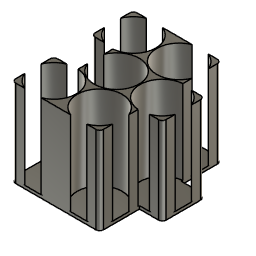
Plate_Holder (Autodesk Fusion 360 design; units mm, degrees)
Autodesk Fusion 360 part; units mm, degrees
note: some values were not read from the file. Set by a fixed rule: which sketch regions a step uses.
sketch "Sketch4" plane through (0, 0, 0) normal (0, 0, 1) x (1, 0, 0)
  circle A0 centre (-30.1021, 33.9333) radius 30
  circle A1 centre (30.8979, 33.9333) radius 30
  circle A2 centre (0.3979, -19.0667) radius 30
  circle A3 centre (-60.6021, -19.0667) radius 30
  line L0 (-84.1021, 5.9333) -> (-84.1021, 6.9333)
  line L1 (27.3979, -43.0667) -> (26.9, -43.0667)
  circle A4 centre (0.3979, 86.9333) radius 30
  circle A5 centre (-60.6021, 86.9333) radius 30
  line L2 (-88.6021, 114.9333) -> (58.8979, 114.9333)
  line L3 (58.8979, 114.9333) -> (58.8979, -47.0667)
  line L4 (58.8979, -47.0667) -> (-88.6021, -47.0667)
  line L5 (-88.6021, -47.0667) -> (-88.6021, 114.9333)
  line L6 (-88.6021, 58.9333) -> (-58.1021, 58.9333)
  line L7 (-58.1021, 58.9333) -> (-58.1021, 8.9333)
  line L8 (-58.1021, 8.9333) -> (-88.6021, 8.9333)
  line L9 (-88.6021, 8.9333) -> (-88.6021, 58.9333)
  line L10 (58.8979, 61.9333) -> (28.3979, 61.9333)
  line L11 (28.3979, 61.9333) -> (28.3979, 114.9333)
  line L12 (28.3979, 114.9333) -> (58.8979, 114.9333)
  line L13 (58.8979, 114.9333) -> (58.8979, 61.9333)
  line L14 (58.8979, 5.9333) -> (28.3979, 5.9333)
  line L15 (28.3979, 5.9333) -> (28.3979, -47.0667)
  line L16 (28.3979, -47.0667) -> (58.8979, -47.0667)
  line L17 (58.8979, -47.0667) -> (58.8979, 5.9333)
  dimension "d15" = 60
  dimension "d16" = 60
  dimension "d17" = 60
  dimension "d18" = 60
  dimension "d19" = 61
  dimension "d23" = 61
  dimension "d24" = 30.5
  dimension "d25" = 53
  dimension "d46" = 60
  dimension "d47" = 60
  dimension "d48" = 61
  dimension "d49" = 53
  dimension "d50" = 30.5
  dimension "d53" = 28
  dimension "d54" = 28
  dimension "d55" = 28
  dimension "d56" = 28
  dimension "d57" = 28
  dimension "d58" = 28
  dimension "d59" = 28
  dimension "d60" = 28
  dimension "d61" = 28
  dimension "d62" = 28
  dimension "d63" = 28
  dimension "d64" = 28
  constraint vertical L0
  constraint horizontal L1
  constraint horizontal L2
  constraint vertical L3
  constraint horizontal L4
  constraint vertical L5
  constraint horizontal L6
  constraint vertical L7
  constraint horizontal L8
  constraint vertical L9
  constraint coincident L5 L6.start
  constraint horizontal L10
  constraint vertical L11
  constraint horizontal L12
  constraint vertical L13
  constraint coincident L2 L11.end
  constraint coincident L3 L10.start
  constraint horizontal L14
  constraint vertical L15
  constraint horizontal L16
  constraint vertical L17
  constraint coincident L4 L15.end
  constraint coincident L3 L14.start
  measures "d15" diameter of A3
  measures "d16" diameter of A2
  measures "d17" diameter of A1
  measures "d18" diameter of A0
  measures "d19" distance of A0.centre A1.centre
  measures "d23" horizontal distance of A2.centre A3.centre
  measures "d24" horizontal distance of A1.centre A2.centre
  measures "d25" vertical distance of A1.centre A2.centre
  measures "d46" diameter of A5
  measures "d47" diameter of A4
  measures "d48" distance of A4.centre A5.centre
  measures "d49" vertical distance of A1.centre A4.centre
  measures "d50" horizontal distance of A1.centre A4.centre
  measures "d53" distance of A2.centre L4
  measures "d54" distance of A4.centre L2
  measures "d55" distance of A5.centre L5
  measures "d56" distance of A3.centre L5
  measures "d57" distance of A1.centre L3
  measures "d58" distance of A5.centre L6
  measures "d59" distance of A0.centre L7
  measures "d60" distance of A3.centre L8
  measures "d61" distance of A4.centre L11
  measures "d62" distance of A1.centre L10
  measures "d63" distance of A2.centre L15
  measures "d64" distance of A1.centre L14
extrude "Extrude6" add sketch "Sketch4" along normal blind 4 contours A0 L7 | A0 A1 A2 A3 A4 A5 L2 L4 L7 L11 L15 | A5 L2 L5 L6 L7 | A3 L4 L5 L7 L8 | A5 L5 L6 | A3 L5 L8 | A5 L2 L5 | A4 L2 L11 | A3 L4 L5 | A2 L4 L15 | A4 L2 L11 | A2 L4 L15 | A1 L3 L10 L11 L14 L15 | A1 L3 L10 | A1 L3 L14 picked at (-22.751, 30.3432)
extrude "Extrude7" add sketch "Sketch4" along normal blind 116 contours A0 A1 A2 A3 A4 A5 L2 L4 L7 L11 L15 | A5 L5 L6 | A3 L5 L8 | A5 L2 L5 | A3 L4 L5 | A4 L2 L11 | A2 L4 L15 | A1 L3 L10 | A1 L3 L14 picked at (22.8223, 111.3226) picked at (22.8223, -43.4561)
fillet "Fillet1" radius 5 8 edges at (28.3979, -47.0667, 58) (58.8979, 5.9333, 58) (58.8979, 61.9333, 58) (28.3979, 114.9333, 58) (-88.6021, 114.9333, 58) (-88.6021, 58.9333, 58) (-88.6021, 8.9333, 58) (-88.6021, -47.0667, 58)
